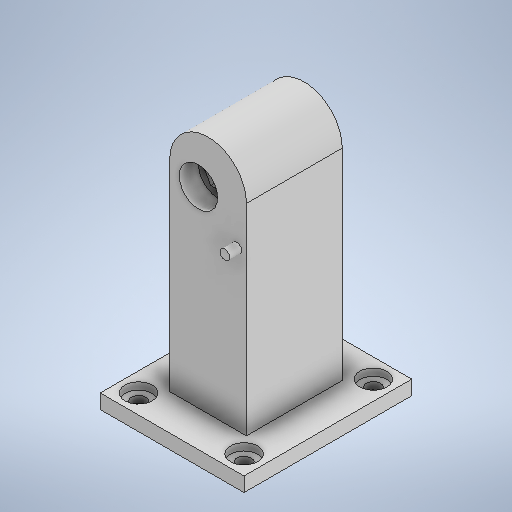
# Autodesk Inventor part: body-2
Saved by Autodesk Inventor 2025 (Build 290162000, 162)
## iProperties
Created: 2026-01-27
Part Number: body-2
Material: 一般
Document SubType Name: Modeling
Designer: mahhy
Density: 1 g/cm^3
Appearance: 既定
Author: mahhy
## iProperties of the stored document body-2_3D プリント.ipt
Created: 2026-01-28
Part Number: body-2_3D プリント
Material: 一般
Document SubType Name: Modeling
Designer: mahhy
Density: 1 g/cm^3
Appearance: 既定
Author: mahhy
Autodesk Inventor part; units mm, degrees
ref_plane "YZ Plane" through (0, 0, 0) normal (1, 0, 0) x (0, 1, 0)
ref_plane "XZ Plane" through (0, 0, 0) normal (0, 1, 0) x (-1, 0, 0)
ref_plane "XY Plane" through (0, 0, 0) normal (0, 0, 1) x (1, 0, 0)
sketch "底面" plane through (0, 0, 0) normal (0, 1, 0) x (-1, 0, 0)
  line L0 (0, 0) -> (-16, 0)
  line L1 (-16, 0) -> (-16, -20)
  line L2 (-16, -20) -> (0, -20)
  line L3 (0, -20) -> (0, 0)
  dimension "d0" = 16
  dimension "d1" = 20
  constraints: 8 end point, 2 parallel, 1 horizontal, 1 perpendicular
  measures "d0" distance of L2.end L1.end
  measures "d1" distance of L1.end L0.end
extrude "本体" add sketch "底面" along normal blind 50
sketch "ねじ穴スケッチ" plane through (0, 0, 0) normal (0, 0, 1) x (1, 0, 0)
  circle A0 centre (6, 40) radius 1.45
  line L0 (0, 50) -> (16, 50) projected
  line L1 (16, 0) -> (16, 50) projected
  point P0 (0, 0)
  dimension "d6" = 10
  dimension "d9" = 2.9
  dimension "d17" = 10
  constraints: 1 centre point
  measures "d6" distance from line of L0 A0.centre
  measures "d9" diameter of A0
  measures "d17" distance from line of L1 A0.centre
extrude "ねじ穴" cut sketch "ねじ穴スケッチ" against normal blind 10
sketch "接合部スケッチ" plane through (0, 0, 0) normal (0, 0, 1) x (1, 0, 0)
  circle A0 centre (6, 40) radius 1.45 projected
  circle A1 centre (6, 40) radius 4
  point P0 (0, 0)
  dimension "d10" = 8
  constraints: 1 centre point, 1 coincident
  measures "d10" diameter of A1
extrude "接合部" cut sketch "接合部スケッチ" against normal blind 4
sketch "スケッチ4" plane through (6, 40, -4) normal (0, 0, 1) x (1, 0, 0)
  line L0 (2.875, 0) -> (1.4375, -2.4898)
  line L1 (1.4375, -2.4898) -> (-1.4375, -2.4898)
  line L2 (-1.4375, -2.4898) -> (-2.875, 0)
  line L3 (-2.875, 0) -> (-1.4375, 2.4898)
  line L4 (-1.4375, 2.4898) -> (1.4375, 2.4898)
  line L5 (1.4375, 2.4898) -> (2.875, 0)
  circle A0 centre (0, 0) radius 1.45 projected
  point P0 (-6, -40)
  point P1 (0, 2.4898)
  dimension "d13" = 2.875
  dimension "d14" = 5.75
  constraints: 12 end point, 1 coincident, 1 midpoint, 1 vertical alignment, 13 other
  measures "d13" distance of L3.end L4.end
  measures "d14" distance of L0.start L2.end
extrude "ナット穴" cut sketch "スケッチ4" against normal blind 2.4
fillet "フィレット1" radius 8 2 edges at (16, 50, -10) (0, 50, -10)
sketch "スケッチ5" plane through (0, 0, 0) normal (0, -1, 0) x (1, 0, 0)
  line L0 (23, 7.5) -> (-7, 7.5)
  line L1 (-7, 7.5) -> (-7, -27.5)
  line L2 (-7, -27.5) -> (23, -27.5)
  line L3 (23, -27.5) -> (23, 7.5)
  line L4 (0, 0) -> (16, 0) projected
  line L5 (16, 0) -> (16, -20) projected
  line L6 (0, -20) -> (0, 0) projected
  line L7 (16, -20) -> (0, -20) projected
  line L8 (0, 0) -> (16, 0) projected
  line L9 (16, 0) -> (16, -20) projected
  point P0 (8, 7.5)
  point P1 (8, 0)
  point P2 (23, -10)
  point P3 (16, -10)
  dimension "d42" = 30
  dimension "d43" = 35
  constraints: 8 end point, 4 midpoint, 2 parallel, 1 horizontal, 1 horizontal alignment, 1 perpendicular, 1 vertical alignment
  measures "d42" distance of L0.start L0.end
  measures "d43" distance of L2.end L0.start
extrude "足場" add sketch "スケッチ5" along normal blind 3 contours L3 L2 L1 L0 | L4 L5 L7 L6
sketch "スケッチ6" plane through (8, 42, 0) normal (0, 0, 1) x (1, 0, 0)
  circle A0 centre (6, -9) radius 1
  line L0 (15, -42) -> (-15, -42) projected
  line L1 (-8, -42) -> (-8, 0) projected
  line L2 (8, -42) -> (8, 0) projected
  dimension "d25" = 2
  dimension "d26" = 33
  dimension "d31" = 2
  constraints: 1 centre point
  measures "d25" diameter of A0
  measures "d26" distance from line of L0 A0.centre
  measures "d31" distance from line of L2 A0.centre
extrude "ストッパー" add sketch "スケッチ6" along normal blind 2.5
sketch "スケッチ7" plane through (0, -3, 0) normal (0, -1, 0) x (1, 0, 0)
  circle A0 centre (-3, 3.5) radius 1.5
  circle A1 centre (19, 3.5) radius 1.5
  circle A2 centre (19, -23.5) radius 1.5
  circle A3 centre (-3, -23.5) radius 1.5
  line L0 (-7, 7.5) -> (-7, -27.5) projected
  line L1 (23, 7.5) -> (-7, 7.5) projected
  line L2 (23, -27.5) -> (23, 7.5) projected
  line L3 (-7, -27.5) -> (23, -27.5) projected
  dimension "d32" = 3
  dimension "d33" = 3
  dimension "d34" = 3
  dimension "d35" = 3
  dimension "d36" = 4
  dimension "d37" = 4
  dimension "d38" = 4
  dimension "d39" = 4
  constraints: 4 centre point, 2 horizontal alignment, 2 vertical alignment
  measures "d32" diameter of A0
  measures "d33" diameter of A1
  measures "d34" diameter of A2
  measures "d35" diameter of A3
  measures "d36" distance from line of L0 A0.centre
  measures "d37" distance from line of L1 A0.centre
  measures "d38" distance from line of L2 A1.centre
  measures "d39" distance from line of L3 A3.centre
extrude "押し出し7" cut sketch "スケッチ7" against normal through all contours A0 | A1 | A2 | A3
sketch "スケッチ8" plane through (0, 0, 0) normal (0, 1, 0) x (1, 0, 0)
  circle A0 centre (-3, 23.5) radius 1.5 projected
  circle A1 centre (-3, 23.5) radius 2.85
  circle A2 centre (19, 23.5) radius 2.85
  circle A3 centre (-3, -3.5) radius 2.85
  circle A4 centre (19, -3.5) radius 2.85
  circle A5 centre (19, 23.5) radius 1.5 projected
  circle A6 centre (19, -3.5) radius 1.5 projected
  circle A7 centre (-3, -3.5) radius 1.5 projected
  point P0 (0, 0)
  dimension "d44" = 5.7
  dimension "d45" = 5.7
  dimension "d46" = 5.7
  dimension "d47" = 5.7
  constraints: 4 centre point, 3 concentric, 1 coincident
  measures "d44" diameter of A1
  measures "d45" diameter of A2
  measures "d46" diameter of A3
  measures "d47" diameter of A4
extrude "ネジ溝" cut sketch "スケッチ8" against normal blind 1.5
equation "\"d17\" = d6"
equation "\"d37\" = d36"
equation "\"d38\" = d36"
equation "\"d39\" = d36"
equation "\"d45\" = d44"
equation "\"d46\" = d44"
equation "\"d47\" = d44"
